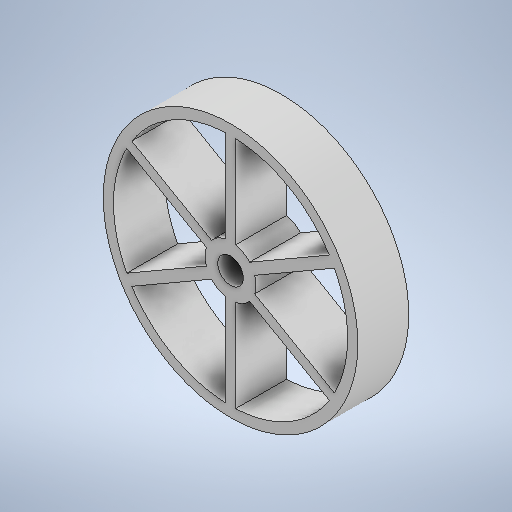
# Autodesk Inventor part: Wheel-D50
Saved by Autodesk Inventor 2025 (Build 290162000, 162)
## iProperties
Created: 2025-07-17
Part Number: Wheel-D50
Material: 一般
Document SubType Name: Modeling
Designer: daisuke
Density: 1 g/cm^3
Appearance: 既定
Author: daisuke
Autodesk Inventor part; units mm, degrees
ref_plane "YZ Plane" through (0, 0, 0) normal (1, 0, 0) x (0, 1, 0)
ref_plane "XZ Plane" through (0, 0, 0) normal (0, 1, 0) x (-1, 0, 0)
ref_plane "XY Plane" through (0, 0, 0) normal (0, 0, 1) x (1, 0, 0)
sketch "スケッチ1" plane through (0, 0, 0) normal (0, 0, 1) x (1, 0, 0)
  circle A0 centre (0, 0) radius 25
  circle A1 centre (0, 0) radius 23
  circle A2 centre (0, 0) radius 5
  circle A3 centre (0, 0) radius 2.5
  dimension "d0" = 50
  dimension "d1" = 2
  dimension "d2" = 10
  dimension "d3" = 5
  constraints: 4 centre point, 4 coincident
  measures "d0" diameter of A0
  measures "d1" radial gap between concentric circles of A0 A1
  measures "d2" diameter of A2
  measures "d3" diameter of A3
extrude "押し出し1" add sketch "スケッチ1" along normal blind 10
sketch "スケッチ2" plane through (0, 0, 0) normal (0, 0, 1) x (1, 0, 0)
  line L0 (-1, 2.5) -> (1, 2.5)
  line L1 (1, 2.5) -> (1, 23)
  line L2 (1, 23) -> (-1, 23)
  line L3 (-1, 23) -> (-1, 2.5)
  circle A0 centre (0, 0) radius 23 projected
  circle A1 centre (0, 0) radius 2.5 projected
  point P0 (0, 2.5)
  point P1 (-1, 22.9783)
  point P2 (1, 22.9783)
  dimension "d6" = 2
  constraints: 8 end point, 2 parallel, 2 tangent, 1 horizontal, 1 midpoint, 1 perpendicular, 1 vertical alignment
  measures "d6" distance between parallel lines of L3 L1
extrude "押し出し2" add sketch "スケッチ2" along normal blind 10 contours L3 A0 L1 L0 picked at (-0.6667, 9.3261)
pattern_circular "円形状パターン1" count 6 over 360 about axis through (0, 0, -10) along (0, 0, 1) of "押し出し2"
